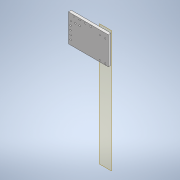
# Autodesk Inventor part: backboard
Saved by Autodesk Inventor 2022 (Build 260153000, 153)
## iProperties
Created: 2021-11-30
Part Number: backboard
Material: Generic
Document SubType Name: Modeling
Designer: efred
Density: 1 g/cm^3
Appearance: Default
Author: efred
Autodesk Inventor part; units mm, degrees
ref_plane "YZ Plane" through (0, 0, 0) normal (1, 0, 0) x (0, 1, 0)
ref_plane "XZ Plane" through (0, 0, 0) normal (0, 1, 0) x (-1, 0, 0)
ref_plane "XY Plane" through (0, 0, 0) normal (0, 0, 1) x (1, 0, 0)
ref_plane "Work Plane1" through (0, 0, 0) normal (0, 0, 1) x (1, 0, 0)
sketch "Sketch1" plane through (0, 0, 0) normal (0, 0, 1) x (1, 0, 0)
  line L0 (-28.1, 210.2) -> (-28.1, 202.1) construction
  line L1 (-28.1, 202.1) -> (-23.1, 202.1) construction
  line L2 (-23.1, 199.1) -> (-23.1, 202.1) construction
  line L3 (-23.1, 199.1) -> (-123.1, 199.1) construction
  line L4 (-123.1, 199.1) -> (-123.1, 210.2) construction
  line L5 (-28.1, 210.2) -> (-123.1, 210.2) construction
  line L6 (-23.1, -199.1) -> (-23.1, -210.2) construction
  line L7 (-23.1, -210.2) -> (-123.1, -210.2) construction
  line L8 (-123.1, -199.1) -> (-123.1, -210.2) construction
  line L9 (-23.1, -199.1) -> (-123.1, -199.1) construction
  line L10 (23, -210.2) -> (-23, -210.2) construction
  line L11 (-23, -210.2) -> (-23, -202.2) construction
  line L12 (23, -202.2) -> (-23, -202.2) construction
  line L13 (23, -210.2) -> (23, -202.2) construction
  line L14 (28, 202.2) -> (-28, 202.2) construction
  line L15 (-28, 202.2) -> (-28, 210.2) construction
  line L16 (28, 210.2) -> (-28, 210.2) construction
  line L17 (28, 202.2) -> (28, 210.2) construction
  line L18 (7.95, 199) -> (7.95, -199) construction
  line L19 (7.95, -199) -> (-7.95, -199) construction
  line L20 (-7.95, -199) -> (-7.95, 199) construction
  line L21 (-7.95, 199) -> (7.95, 199) construction
  line L22 (-11.95, 199) -> (-11.95, -199) construction
  line L23 (-11.95, -199) -> (-19.95, -199) construction
  line L24 (-19.95, -199) -> (-19.95, 199) construction
  line L25 (-19.95, 199) -> (-11.95, 199) construction
  line L26 (11.95, -199) -> (11.95, 199) construction
  line L27 (11.95, 199) -> (19.95, 199) construction
  line L28 (19.95, 199) -> (19.95, -199) construction
  line L29 (19.95, -199) -> (11.95, -199) construction
  line L30 (-123.1, 210.2) -> (19.95, 210.2)
  line L31 (19.95, 210.2) -> (19.95, 110.2)
  line L32 (19.95, 110.2) -> (-123.1, 110.2)
  line L33 (-123.1, 110.2) -> (-123.1, 210.2)
  circle A0 centre (-9.95, 115.2) radius 2.15
  circle A1 centre (9.95, 115.2) radius 2.15
  circle A2 centre (9.95, 194) radius 2.15
  circle A3 centre (-9.95, 194) radius 2.15
  line L34 (-11.95, 155.8556) -> (-7.95, 155.8556) construction
  line L35 (7.95, 155.8556) -> (11.95, 155.8556) construction
  line L36 (-9.95, 155.8556) -> (-9.95, 110.2) construction
  line L37 (9.95, 155.8556) -> (9.95, 110.2) construction
  line L38 (-89.6001, 199.1) -> (-89.6001, 210.2) construction
  line L39 (-89.6001, 204.65) -> (-123.1, 204.65) construction
  circle A4 centre (-103.1, 204.65) radius 2.65
  circle A5 centre (-83.1, 204.65) radius 2.65
  circle A6 centre (-63.1, 204.65) radius 2.65
  circle A7 centre (-43.1, 204.65) radius 2.65
  point P0 (0, 0)
extrude "Extrusion1" add sketch "Sketch1" along normal blind 10
sketch "Sketch2" plane through (0, 0, 0) normal (0, 0, -1) x (-1, 0, 0)
  circle A0 centre (83.1, 186.5) radius 2.65 construction
  circle A1 centre (98.1, 186.5) radius 2.65 construction
  circle A2 centre (113.1, 186.5) radius 2.65 construction
  circle A3 centre (83.1, 186.5) radius 2.5
  circle A4 centre (98.1, 186.5) radius 2.5
  circle A5 centre (113.1, 186.5) radius 2.5
  point P0 (0, 0)
  dimension "d20" = 5
  dimension "d21" = 5
  dimension "d22" = 5
  constraints: 3 centre point, 3 coincident
  measures "d20" diameter of A3
  measures "d21" diameter of A4
  measures "d22" diameter of A5
extrude "Extrusion2" cut sketch "Sketch2" against normal through all
sketch "Sketch3" plane through (0, 0, 10) normal (0, 0, 1) x (1, 0, 0)
  circle A0 centre (-115.6, 141.5) radius 2.65 construction
  circle A1 centre (-115.6, 156.5) radius 2.65 construction
  circle A2 centre (-115.6, 126.5) radius 2.65 construction
  circle A3 centre (-115.6, 171.5) radius 2.65 construction
  arc A4 (-111.2, 191.1249) -> (-111.2, 181.8751) centre (-113.1, 186.5) ccw construction
  line L0 (-111.2, 264.8) -> (-111.2, 191.1249) construction
  line L1 (-111.2, 264.8) -> (-223.2, 264.8) construction
  line L2 (-223.2, 105.1) -> (-223.2, 264.8) construction
  line L3 (-223.2, 105.1) -> (-111.2, 105.1) construction
  line L4 (-111.2, 181.8751) -> (-111.2, 105.1) construction
  circle A5 centre (-115.6, 171.5) radius 2.5
  circle A6 centre (-115.6, 156.5) radius 2.5
  circle A7 centre (-115.6, 141.5) radius 2.5
  circle A8 centre (-115.6, 126.5) radius 2.5
  point P0 (0, 0)
  dimension "d25" = 5
  dimension "d28" = 15
  constraints: 4 centre point, 1 coincident, 1 vertical, 6 other
  measures "d25" diameter of A5
  measures "d28" distance of A5.centre A6.centre
extrude "Extrusion3" cut sketch "Sketch3" against normal through all
equation "\"d2\" = d1"
equation "\"d3\" = d1"
equation "\"d4\" = d1"
equation "\"d6\" = d5"
equation "\"d7\" = d5"
equation "\"d8\" = d5"
equation "\"d1\" = 4.3"
equation "\"d5\" = 5"
body "Solid1"
